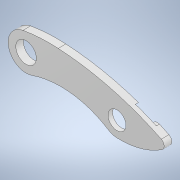
# Autodesk Inventor part: 揺動節
Saved by Autodesk Inventor 2022.2 (Build 262287000, 287)
## iProperties
Created: 2022-01-09
Part Number: 揺動節
Material: Aluminum 2014-T6
Document SubType Name: Modeling
Designer: acps
Density: 2.78927 g/cm^3
Appearance: Satin
Author: acps
Autodesk Inventor part; units mm, degrees
ref_plane "YZ Plane" through (0, 0, 0) normal (1, 0, 0) x (0, 1, 0)
ref_plane "XZ Plane" through (0, 0, 0) normal (0, 1, 0) x (-1, 0, 0)
ref_plane "XY Plane" through (0, 0, 0) normal (0, 0, 1) x (1, 0, 0)
sketch "Sketch1" plane through (0, 0, 0) normal (0, 0, 1) x (1, 0, 0)
  line L0 (64.2923, 12.9984) -> (99.9168, 7.8124) construction
  circle A0 centre (64.2923, 12.9984) radius 3 construction
  circle A1 centre (64.2923, 12.9984) radius 4.025
  circle A2 centre (64.2923, 12.9984) radius 7
  arc A3 (102.8654, 13.0378) -> (100.7509, 14.1759) centre (73.379, -39.2168) ccw construction
  arc A4 (96.6891, 2.7545) -> (66.5537, 6.3738) centre (77.8606, -26.7495) ccw
  circle A5 centre (99.9168, 7.8124) radius 2.5 construction
  circle A6 centre (99.9168, 7.8124) radius 3.525
  circle A7 centre (99.9168, 7.8124) radius 6
  line L1 (99.9168, 7.8124) -> (116.9156, -6.1534) construction
  circle A8 centre (116.9156, -6.1534) radius 10 construction
  circle A9 centre (116.9156, -6.1534) radius 7.025 construction
  line L2 (102.8192, 13.0637) -> (121.753, 2.5988) construction
  line L3 (95.3285, 3.9461) -> (109.2685, -12.5971) construction
  line L4 (109.1054, 9.7035) -> (127.2456, -0.3228) construction
  arc A10 (99.6026, 1.8206) -> (117.4793, 6.5976) centre (101.1737, 31.7794) ccw
  arc A11 (117.2714, 10.0728) -> (76.903, 20.6796) centre (70.6772, -85.1374) ccw
  arc A12 (117.4793, 6.5976) -> (117.2714, 10.0728) centre (116.3923, 8.2764) ccw
  line L5 (64.2923, 12.9984) -> (100, 0)
  line L6 (100, 0) -> (116.9156, -6.1534) construction
  arc A13 (113.5757, 11.7941) -> (111.7988, 8.2148) centre (112.7663, 9.9652) ccw
  line L7 (99.9168, 7.8124) -> (79.3942, -0.1137) construction
  circle A14 centre (79.3942, -0.1137) radius 7.025 construction
  circle A15 centre (79.3942, -0.1137) radius 10 construction
  line L8 (77.5476, 9.7143) -> (98.8088, 13.7092) construction
  line L9 (111.7988, 8.2148) -> (116.172, 5.7977)
  line L10 (74.571, 9.2567) -> (105.334, 15.037)
  arc A16 (76.903, 20.6796) -> (63.0922, 19.8948) centre (73.379, -39.2168) ccw
  arc A17 (100.7509, 14.1759) -> (76.903, 20.6796) centre (73.379, -39.2168) ccw construction
  arc A18 (74.571, 9.2567) -> (73.0408, 7.917) centre (74.9404, 7.2911) ccw
  point P0 (0, 0)
  point P1 (89.0424, -2.743)
  point P2 (88.317, -4.6285)
  dimension "d0" = 36
  dimension "d1" = 8.05
  dimension "d2" = 6
  dimension "d3" = 14
  dimension "d4" = 60
  dimension "d5" = 35
  dimension "d8" = 22
  dimension "d10" = 12
  dimension "d11" = 7.05
  dimension "d12" = 20
  dimension "d13" = 14.05
  dimension "d15" = 0.1
  dimension "d16" = 30
  dimension "d17" = 5
  dimension "d18" = 2
  dimension "d19" = 106
  dimension "d21" = 121
  dimension "d46" = 12.9985
  dimension "d47" = 38
  dimension "d48" = 18
  dimension "d50" = 0
  dimension "d51" = 100
  dimension "d52" = 11.72
  dimension "d53" = 2
  dimension "d54" = 4
  dimension "d55" = 22
  dimension "d56" = 14.05
  dimension "d57" = 20
  dimension "d58" = 29.4
  dimension "d59" = 0.1
  dimension "d60" = 2
  constraints: 35 point on circle, 22 end point, 19 centre point, 17 tangent, 10 coincident, 4 point on line, 2 parallel
  measures "d0" distance of L0.start L0.end
  measures "d1" diameter of A1
  measures "d2" diameter of A0
  measures "d3" diameter of A2
  measures "d4" radius of A3
  measures "d5" radius of A4
  measures "d8" distance of L1.start L1.end
  measures "d10" diameter of A7
  measures "d11" diameter of A6
  measures "d12" diameter of A8
  measures "d13" diameter of A9
  measures "d15" distance between parallel lines of L2 L4
  measures "d16" radius of A10
  measures "d17" diameter of A5
  measures "d18" radius of A12
  measures "d19" radius of A11
  measures "d46" vertical distance of point (0, 0) L0.start
  measures "d47" distance of L5.start L5.end
  measures "d48" distance of L5.end L6.end
  measures "d50" vertical distance of point (0, 0) L5.end
  measures "d51" distance of point (0, 0) L5.end
  measures "d52" angle of L5 L0
  measures "d53" radius of A13
  measures "d54" distance of A12.centre A13.centre
  measures "d55" distance of L1.start L7.end
  measures "d56" diameter of A14
  measures "d57" diameter of A15
  measures "d58" angle of L0 L7
  measures "d59" distance between parallel lines of L8 L10
  measures "d60" radius of A18
extrude "Extrusion5" add sketch "Sketch1" against normal blind 3 contours A2 | A2 A16 A11 L10 L5 | L5 A18 A4 A2 | A11 A12 A10 L9 A13
extrude "Extrusion6" add sketch "Sketch1" against normal blind 1.8 contours L10 A11 A13 L9 A10 A7 A4 L5 | L5 A4 A18 | A7
body "Solid3"
